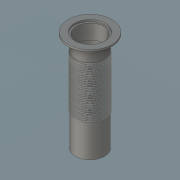
# Autodesk Inventor part: KF50 bellows
Saved by Autodesk Inventor 2018 (Build 220112000, 112)
## iProperties
Created: 2019-01-14
Part Number: KF50 bellows
Material: Generic
Document SubType Name: Modeling
Designer: Admin
Density: 1 g/cm^3
Appearance: Stainless - Brushed
Author: Admin
Autodesk Inventor part; units mm, degrees
ref_plane "YZ Plane" through (0, 0, 0) normal (1, 0, 0) x (0, 1, 0)
ref_plane "XZ Plane" through (0, 0, 0) normal (0, 1, 0) x (-1, 0, 0)
ref_plane "XY Plane" through (0, 0, 0) normal (0, 0, 1) x (1, 0, 0)
sketch "Sketch1" plane through (0, 0, 0) normal (0, 1, 0) x (-1, 0, 0)
  circle A0 centre (0, 0) radius 37.465
  circle A1 centre (0, 0) radius 26.289
  dimension "d0" = 74.93
  dimension "d1" = 52.578
  constraints: 2 centre point, 2 coincident
  measures "d0" diameter of A0
  measures "d1" diameter of A1
extrude "Extrusion1" add sketch "Sketch1" against normal blind 3.048
sketch "Sketch2" plane through (0, -3.048, 0) normal (0, -1, 0) x (1, 0, 0)
  circle A0 centre (0, 0) radius 37.465
  circle A1 centre (0, 0) radius 37.465 projected
  constraints: 1 centre point, 1 coincident, 1 concentric
extrude "Extrusion2" add sketch "Sketch2" along normal blind 6.35 draft -75
sketch "Sketch3" plane through (0, -3.048, 0) normal (0, 1, 0) x (1, 0, 0)
  circle A0 centre (0, 0) radius 23.241
  circle A1 centre (0, 0) radius 26.289 projected
  dimension "d6" = 3.048
  constraints: 1 centre point, 1 coincident
  measures "d6" radial gap between concentric circles of A1 A0
extrude "Extrusion3" cut sketch "Sketch3" against normal up to surface (6.35 mm away) contours A0
sketch "Sketch4" plane through (0, -3.048, 0) normal (0, 1, 0) x (1, 0, 0)
  circle A0 centre (0, 0) radius 23.241
  circle A1 centre (0, 0) radius 23.241 projected
  circle A2 centre (0, 0) radius 25.019
  dimension "d9" = 50.038
  constraints: 2 centre point, 2 coincident, 1 concentric
  measures "d9" diameter of A2
extrude "Extrusion4" add sketch "Sketch4" against normal blind 25.4
sketch "Sketch5" plane through (0, 0, 0) normal (0, 0, 1) x (1, 0, 0)
  line L0 (-25.019, -28.448) -> (25.019, -28.448) projected
  line L1 (25.019, -28.448) -> (25.019, -29.718)
  circle A0 centre (25.019, -29.718) radius 1.27
  line L2 (23.241, -28.448) -> (-23.241, -28.448) projected
  line L3 (23.241, -28.448) -> (112.141, -28.448) construction
  circle A1 centre (25.019, -32.258) radius 1.27
  circle A2 centre (25.019, -34.798) radius 1.27
  circle A3 centre (25.019, -37.338) radius 1.27
  circle A4 centre (25.019, -39.878) radius 1.27
  circle A5 centre (25.019, -42.418) radius 1.27
  circle A6 centre (25.019, -44.958) radius 1.27
  circle A7 centre (25.019, -47.498) radius 1.27
  circle A8 centre (25.019, -50.038) radius 1.27
  circle A9 centre (25.019, -52.578) radius 1.27
  circle A10 centre (25.019, -55.118) radius 1.27
  circle A11 centre (25.019, -57.658) radius 1.27
  circle A12 centre (25.019, -60.198) radius 1.27
  circle A13 centre (25.019, -62.738) radius 1.27
  circle A14 centre (25.019, -65.278) radius 1.27
  circle A15 centre (25.019, -67.818) radius 1.27
  circle A16 centre (25.019, -70.358) radius 1.27
  circle A17 centre (25.019, -72.898) radius 1.27
  circle A18 centre (25.019, -75.438) radius 1.27
  circle A19 centre (25.019, -77.978) radius 1.27
  circle A20 centre (25.019, -80.518) radius 1.27
  circle A21 centre (25.019, -83.058) radius 1.27
  circle A22 centre (25.019, -85.598) radius 1.27
  circle A23 centre (25.019, -88.138) radius 1.27
  circle A24 centre (25.019, -90.678) radius 1.27
  circle A25 centre (25.019, -93.218) radius 1.27
  circle A26 centre (25.019, -95.758) radius 1.27
  circle A27 centre (25.019, -98.298) radius 1.27
  circle A28 centre (25.019, -100.838) radius 1.27
  circle A29 centre (25.019, -103.378) radius 1.27
  circle A30 centre (25.019, -105.918) radius 1.27
  circle A31 centre (25.019, -108.458) radius 1.27
  circle A32 centre (25.019, -110.998) radius 1.27
  circle A33 centre (25.019, -113.538) radius 1.27
  circle A34 centre (25.019, -116.078) radius 1.27
  line L4 (25.019, -28.448) -> (23.495, -28.448)
  line L5 (23.495, -28.448) -> (23.495, -117.348)
  line L6 (23.495, -117.348) -> (25.019, -117.348)
  line L7 (25.019, -117.348) -> (25.019, -28.448)
  line L8 (0, -140.8176) -> (0, 23.4696) projected
  point P0 (0, 0)
  point P1 (25.019, -30.988)
  point P2 (25.019, -33.528)
  point P3 (25.019, -36.068)
  point P4 (25.019, -38.608)
  point P5 (25.019, -41.148)
  point P6 (25.019, -43.688)
  point P7 (25.019, -46.228)
  point P8 (25.019, -48.768)
  point P9 (25.019, -51.308)
  point P10 (25.019, -53.848)
  point P11 (25.019, -56.388)
  point P12 (25.019, -58.928)
  point P13 (25.019, -61.468)
  point P14 (25.019, -64.008)
  point P15 (25.019, -66.548)
  point P16 (25.019, -69.088)
  point P17 (25.019, -71.628)
  point P18 (25.019, -74.168)
  point P19 (25.019, -76.708)
  point P20 (25.019, -79.248)
  point P21 (25.019, -81.788)
  point P22 (25.019, -84.328)
  point P23 (25.019, -86.868)
  point P24 (25.019, -89.408)
  point P25 (25.019, -91.948)
  point P26 (25.019, -94.488)
  point P27 (25.019, -97.028)
  point P28 (25.019, -99.568)
  point P29 (25.019, -102.108)
  point P30 (25.019, -104.648)
  point P31 (25.019, -107.188)
  point P32 (25.019, -109.728)
  point P33 (25.019, -112.268)
  point P34 (25.019, -114.808)
  dimension "d12" = 1.27
  dimension "d17" = 2.54
  dimension "d22" = 1.524
  dimension "d23" = 88.9
  constraints: 36 vertical, 35 vertical alignment, 12 end point, 2 horizontal, 2 parallel, 1 coincident, 1 perpendicular, 138 other
  measures "d12" distance of L0.end L1.end
  measures "d17" distance of point (25.019, -29.718) point (25.019, -32.258)
  measures "d22" distance of L6.end L5.end
  measures "d23" distance of L5.end L4.end
revolve "Revolution1" add sketch "Sketch5" angle 360 about axis through (0, -10, 0) along (0, 1, 0)
sketch "Sketch6" plane through (0, -117.348, 0) normal (0, -1, 0) x (1, 0, 0)
  circle A0 centre (0, 0) radius 23.495
  circle A1 centre (0, 0) radius 23.495 projected
  circle A2 centre (0, 0) radius 25.019
  circle A3 centre (0, 0) radius 25.019 projected
  constraints: 2 centre point, 2 coincident, 2 concentric
extrude "Extrusion5" add sketch "Sketch6" along normal blind 55.372
body "Solid1"
